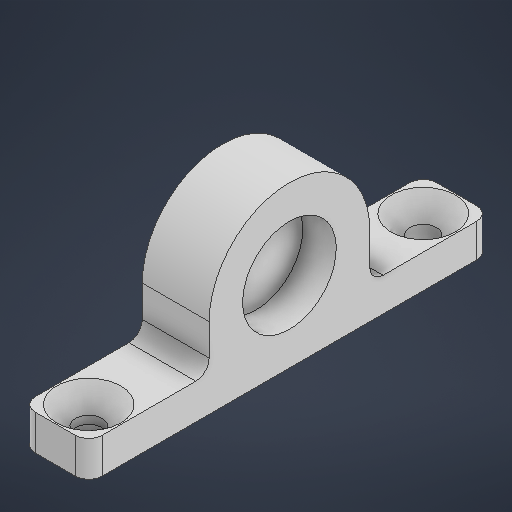
# Autodesk Inventor part: bearing_holder
Saved by Autodesk Inventor 2026.2 (Build 302298000, 298)
## iProperties
Created: 2026-01-17
Part Number: bearing_holder
Material: Generic
Document SubType Name: Modeling
Designer: User
Density: 1 g/cm^3
Appearance: Default
Author: User
Autodesk Inventor part; units mm, degrees
ref_plane "YZ Plane" through (0, 0, 0) normal (1, 0, 0) x (0, 1, 0)
ref_plane "XZ Plane" through (0, 0, 0) normal (0, 1, 0) x (-1, 0, 0)
ref_plane "XY Plane" through (0, 0, 0) normal (0, 0, 1) x (1, 0, 0)
sketch "Sketch1" plane through (0, 0, 0) normal (1, 0, 0) x (0, 1, 0)
  circle A0 centre (0, 0) radius 7
  arc A1 (0, -12) -> (0, 12) centre (0, 0) ccw
  circle A2 centre (0, 0) radius 2.475
  line L0 (-12, -30) -> (-12, 29.9986)
  line L1 (-6.7144, 29.9986) -> (-12, 29.9986)
  line L2 (-12, -30) -> (-7, -30)
  line L3 (-7, -30) -> (-7, -12)
  line L4 (0, -12) -> (-7, -12)
  line L5 (0, 12) -> (-6.7144, 12)
  line L6 (-6.7144, 12) -> (-6.7144, 29.9986)
  point P0 (-7, 0)
  dimension "d0" = 14
  dimension "d1" = 30
  dimension "d2" = 30
  dimension "d4" = 5
  dimension "d5" = 4.95
  dimension "d22" = 5
  constraints: 14 end point, 2 centre point, 2 coincident, 2 horizontal, 2 perpendicular, 2 point on circle, 2 tangent, 2 vertical, 1 horizontal alignment, 1 parallel, 2 other
  measures "d1" distance of point (-7, 0) L2.end
  measures "d2" distance of point (-7, 0) L1.start
  measures "d5" diameter of A2
  measures "d22" distance from line of point (-7, 0) L0
extrude "Extrusion1" add sketch "Sketch1" along normal blind 5 contours A0 | A2
extrude "Extrusion2" add sketch "Sketch1" along normal blind 10 contours L4 L3 L2 L0 L1 L6 L5 A1
sketch "Sketch3" plane through (0, -7, -12) normal (0, 1, 0) x (1, 0, 0)
  circle A0 centre (5, 13) radius 2
  line L0 (0, 18) -> (10, 18) projected
  point P0 (0, -12)
  point P1 (5, 18)
  dimension "d26" = 4
  dimension "d27" = 0
  dimension "d28" = 5
  constraints: 1 centre point, 1 midpoint
  measures "d26" diameter of A0
  measures "d27" horizontal distance of point (5, 18) A0.centre
  measures "d28" distance from line of L0 A0.centre
extrude "Extrusion4" cut sketch "Sketch3" against normal blind 10
chamfer "Chamfer4" distance 2.8 angle 45 1 edges at (3, -7, -25)
fillet "Fillet2" radius 2 2 edges at (10, -9.5, -30) (0, -9.5, -30)
sketch "Sketch4" plane through (0, -6.7144, 29.9986) normal (0, 1, 0) x (1, 0, 0)
  circle A0 centre (5, 5) radius 2
  line L0 (0, 0) -> (10, 0) projected
  point P0 (0, 29.9986)
  point P1 (5, 0)
  dimension "d35" = 4
  dimension "d36" = 0
  dimension "d37" = 5
  constraints: 1 centre point, 1 midpoint
  measures "d35" diameter of A0
  measures "d36" horizontal distance of point (5, 0) A0.centre
  measures "d37" distance from line of L0 A0.centre
extrude "Extrusion5" cut sketch "Sketch4" against normal blind 4
chamfer "Chamfer5" distance 2.8 angle 45 1 edges at (3, -6.7144, 24.9986)
fillet "Fillet3" radius 2 4 edges at (0, -9.3572, 29.9986) (10, -9.3572, 29.9986) (5, -6.7144, 12) (5, -7, -12)
equation "\"d38\" = d35"
body "Solid1"
